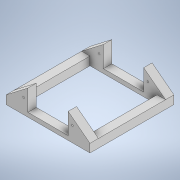
# Autodesk Inventor part: MotorMountForPrograming
Saved by Autodesk Inventor 2020 (Build 240168000, 168)
## iProperties
Created: 2023-01-29
Part Number: MotorMountForPrograming
Material: Generic
Document SubType Name: Modeling
Designer: legoo
Density: 1 g/cm^3
Appearance: Default
Author: legoo
Autodesk Inventor part; units mm, degrees
ref_plane "YZ Plane" through (0, 0, 0) normal (1, 0, 0) x (0, 1, 0)
ref_plane "XZ Plane" through (0, 0, 0) normal (0, 1, 0) x (-1, 0, 0)
ref_plane "XY Plane" through (0, 0, 0) normal (0, 0, 1) x (1, 0, 0)
sketch "Sketch1" plane through (0, 0, 0) normal (0, 1, 0) x (-1, 0, 0)
  line L0 (0, 0) -> (-50, 0)
  line L1 (-50, 0) -> (-50, -50)
  line L2 (-50, -50) -> (0, -50)
  line L3 (0, -50) -> (0, 0)
  line L4 (-5, -5) -> (-45, -5)
  line L5 (-45, -5) -> (-45, -45)
  line L6 (-45, -45) -> (-5, -45)
  line L7 (-5, -45) -> (-5, -5)
  dimension "d0" = 50
  dimension "d1" = 50
  dimension "d2" = 5
  constraints: 16 end point, 4 parallel, 2 perpendicular, 1 horizontal, 3 other
  measures "d0" distance of L2.end L0.start
  measures "d1" distance of L1.end L2.end
  measures "d2" distance between parallel lines of L7 L3
extrude "Extrusion1" add sketch "Sketch1" along normal blind 5
sketch "Sketch2" plane through (0, 0, 0) normal (0, 0, 1) x (1, 0, 0)
  line L0 (0, 5) -> (50, 5) projected
  line L1 (13, 5) -> (37, 5)
  line L2 (37, 5) -> (37, 2.5)
  line L3 (37, 2.5) -> (13, 2.5)
  line L4 (13, 2.5) -> (13, 5)
  line L5 (0, 0) -> (50, 0) projected
  line L6 (0, 0) -> (0, 5) projected
  dimension "d5" = 24
  dimension "d6" = 2.5
  dimension "d7" = 13
  constraints: 8 end point, 2 parallel, 1 horizontal, 1 perpendicular, 1 point on line
  measures "d5" distance of L2.end L3.end
  measures "d6" distance between parallel lines of L5 L3
  measures "d7" distance between parallel lines of L6 L4
extrude "Extrusion2" cut sketch "Sketch2" against normal through all
sketch "Sketch3" plane through (0, 0, 0) normal (0, 0, 1) x (1, 0, 0)
  line L0 (13, 2.5) -> (13, 5) projected
  line L1 (13, 5) -> (13, 15)
  line L2 (13, 5) -> (0, 5) projected
  line L3 (13, 15) -> (0, 5)
  line L4 (37, 5) -> (37, 2.5) projected
  line L5 (37, 5) -> (37, 15)
  line L6 (50, 5) -> (37, 5) projected
  line L7 (37, 15) -> (50, 5)
  point P0 (0, 0)
  dimension "d10" = 10
  dimension "d11" = 10
  constraints: 8 end point, 2 vertical
  measures "d10" distance of L0.end L1.end
  measures "d11" distance of L4.start L5.end
extrude "Extrusion3" add sketch "Sketch3" against normal blind 5
sketch "Sketch4" plane through (50, 0, -50) normal (0, 0, -1) x (-1, 0, 0)
  line L0 (50, 5) -> (37, 15) projected
  line L1 (37, 15) -> (37, 2.5) projected
  line L2 (13, 15) -> (0, 5) projected
  line L3 (13, 2.5) -> (13, 15) projected
  line L4 (0, 5) -> (13, 15)
  line L5 (13, 5) -> (5, 5) projected
  line L6 (13, 15) -> (13, 5)
  line L7 (0, 5) -> (13, 5) projected
  line L8 (13, 5) -> (0, 5)
  line L9 (50, 5) -> (45, 5) projected
  line L10 (50, 5) -> (37, 15)
  line L11 (45, 5) -> (37, 5) projected
  line L12 (37, 15) -> (37, 5)
  line L13 (37, 5) -> (50, 5)
  point P0 (50, 0)
  constraints: 12 end point, 3 perpendicular, 1 collinear, 1 point on line
extrude "Extrusion4" add sketch "Sketch4" against normal blind 5
sketch "Sketch5" plane through (50, 0, -50) normal (0, 0, -1) x (-1, 0, 0)
  circle A0 centre (39.5, 9) radius 0.5
  circle A1 centre (10.5, 9) radius 0.5
  line L0 (37, 2.5) -> (13, 2.5) projected
  line L1 (37, 15) -> (37, 2.5) projected
  line L2 (13, 2.5) -> (13, 15) projected
  point P0 (50, 0)
  dimension "d16" = 6.5
  dimension "d17" = 6.5
  dimension "d18" = 1
  dimension "d19" = 1
  dimension "d20" = 2.5
  dimension "d21" = 2.5
  constraints: 2 centre point
  measures "d16" distance from line of L0 A0.centre
  measures "d17" distance from line of L0 A1.centre
  measures "d18" diameter of A1
  measures "d19" diameter of A0
  measures "d20" distance from line of A0.centre L1
  measures "d21" distance from line of L2 A1.centre
sketch "Sketch6" plane through (50, 0, -50) normal (0, 0, -1) x (-1, 0, 0)
  point P0 (50, 0)
extrude "Extrusion5" cut sketch "Sketch5" against normal through all
body "Solid1"
